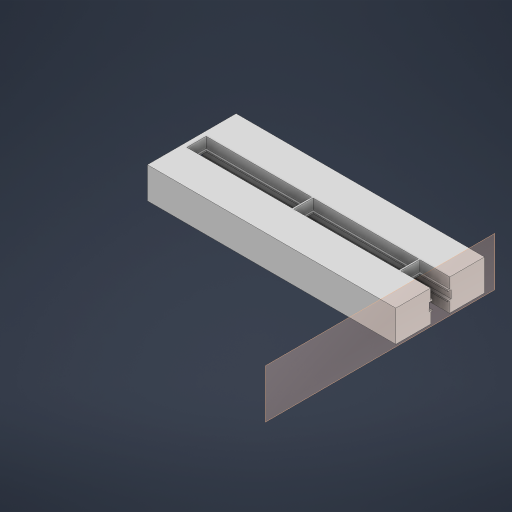
# Autodesk Inventor part: magnets nest half
Saved by Autodesk Inventor 2023 (Build 270158000, 158)
## iProperties
Created: 2023-08-23
Part Number: magnets nest half
Material: Generic
Document SubType Name: Modeling
Designer: f1a51
Density: 1 g/cm^3
Appearance: Default
Author: f1a51
Autodesk Inventor part; units mm, degrees
ref_plane "XZ Plane" through (0, 0, 0) normal (0, 1, 0) x (-1, 0, 0)
ref_plane "XY Plane" through (0, 0, 0) normal (0, 0, 1) x (1, 0, 0)
sketch "Sketch1" plane through (0, 0, 0) normal (1, 0, 0) x (0, 1, 0)
  line L0 (-6, -6) -> (6, -6)
  line L1 (6, -6) -> (6, 6)
  line L2 (6, 6) -> (-6, 6)
  line L3 (-6, 6) -> (-6, -6)
  line L4 (-6, -6) -> (6, 6) construction
  line L5 (6, -6) -> (-6, 6) construction
  line L6 (11, -40) -> (6, -40)
  line L7 (6, -40) -> (6, 40)
  line L8 (6, 40) -> (11, 40)
  line L9 (11, 40) -> (11, -40)
  line L10 (11, -40) -> (6, 40) construction
  line L11 (6, -40) -> (11, 40) construction
  line L12 (0, 24.7928) -> (0, 31.3359)
  line L13 (-11, -40) -> (-6, -40)
  line L14 (-6, -40) -> (-6, 40)
  line L15 (-6, 40) -> (-11, 40)
  line L16 (-11, 40) -> (-11, -40)
  line L17 (-11, -40) -> (-6, 40) construction
  line L18 (-6, -40) -> (-11, 40) construction
  line L19 (6, -21.3242) -> (2, -21.3242)
  line L20 (2, -21.3242) -> (2, -28.3242)
  line L21 (2, -28.3242) -> (6, -28.3242)
  line L22 (6, -28.3242) -> (6, -21.3242)
  line L23 (-6, -21.3242) -> (-2, -21.3242)
  line L24 (-2, -21.3242) -> (-2, -28.3242)
  line L25 (-2, -28.3242) -> (-6, -28.3242)
  line L26 (0, 0) -> (26.7242, 0)
  line L27 (6, 21.3242) -> (2, 21.3242)
  line L28 (2, 21.3242) -> (2, 28.3242)
  line L29 (2, 28.3242) -> (6, 28.3242)
  line L30 (-6, 21.3242) -> (-2, 21.3242)
  line L31 (-2, 21.3242) -> (-2, 28.3242)
  line L32 (-2, 28.3242) -> (-6, 28.3242)
  point P0 (8.5, 0)
  dimension "d0" = 12
  dimension "d1" = 12
  dimension "d2" = 80
  dimension "d3" = 5
  dimension "d4" = 0
  dimension "d5" = 0
  dimension "d6" = 4
  dimension "d7" = 7
  constraints: 66 end point, 16 symmetric about line, 6 parallel, 4 horizontal, 4 midpoint, 3 perpendicular, 1 point on line, 1 vertical
  measures "d0" distance of L1.end L2.end
  measures "d1" distance of L0.end L1.end
  measures "d2" distance of L8.end L6.start
  measures "d3" distance of L7.end L8.end
  measures "d4" vertical distance of L26.start point (8.5, 0)
  measures "d5" distance between parallel lines of L1 L7
  measures "d6" distance of L21.end L20.end
  measures "d7" distance of L20.end L19.end
extrude "Extrusion1" add sketch "Sketch1" along normal blind 290 contours L3 L2 L1 L0 | L1 L26 L9 L6 L7 | L1 L7 L8 L9 L26
sketch "Sketch3" plane through (0, 6, -40) normal (0, -1, 0) x (1, 0, 0)
  line L0 (290, 34) -> (290, 0) projected
  line L1 (290, 0) -> (290, 13.5)
  line L2 (290, 13.5) -> (288, 13.5)
  line L3 (288, 13.5) -> (288, 20.5)
  line L4 (288, 20.5) -> (248, 20.5)
  line L5 (248, 20.5) -> (248, 13.5)
  line L6 (248, 13.5) -> (288, 13.5)
  line L7 (248, 20.5) -> (247, 20.5)
  line L8 (247, 13.5) -> (247, 20.5)
  line L9 (247, 20.5) -> (207, 20.5)
  line L10 (207, 20.5) -> (207, 13.5)
  line L11 (207, 13.5) -> (247, 13.5)
  line L12 (207, 20.5) -> (206, 20.5)
  line L13 (206, 13.5) -> (206, 20.5)
  line L14 (206, 20.5) -> (166, 20.5)
  line L15 (166, 20.5) -> (166, 13.5)
  line L16 (166, 13.5) -> (206, 13.5)
  line L17 (166, 20.5) -> (165, 20.5)
  line L18 (165, 13.5) -> (165, 20.5)
  line L19 (165, 20.5) -> (125, 20.5)
  line L20 (125, 20.5) -> (125, 13.5)
  line L21 (125, 13.5) -> (165, 13.5)
  line L22 (125, 20.5) -> (124, 20.5)
  line L23 (124, 13.5) -> (124, 20.5)
  line L24 (124, 20.5) -> (84, 20.5)
  line L25 (84, 20.5) -> (84, 13.5)
  line L26 (84, 13.5) -> (124, 13.5)
  line L27 (84, 20.5) -> (83, 20.5)
  line L28 (83, 13.5) -> (83, 20.5)
  line L29 (83, 20.5) -> (43, 20.5)
  line L30 (43, 20.5) -> (43, 13.5)
  line L31 (43, 13.5) -> (83, 13.5)
  line L32 (43, 20.5) -> (42, 20.5)
  line L33 (42, 13.5) -> (42, 20.5)
  line L34 (42, 20.5) -> (2, 20.5)
  line L35 (2, 20.5) -> (2, 13.5)
  line L36 (2, 13.5) -> (42, 13.5)
  line L37 (0, 0) -> (290, 0) projected
  line L38 (0, 34) -> (290, 34) projected
  line L39 (0, 34) -> (0, 0) projected
  point P0 (0, 40)
  dimension "d15" = 13.5
  constraints: 72 end point, 15 perpendicular, 7 horizontal, 2 point on line
  measures "d15" distance of L0.end L1.end
extrude "Extrusion2" add sketch "Sketch3" along normal blind 12 separate body
sketch "Sketch4" plane through (0, 6, -40) normal (-1, 0, 0) x (0, 0, 1)
  line L0 (13.5, 0) -> (13.5, -12) projected
  line L1 (13.5, -12) -> (13.5, -8)
  line L2 (13.5, -8) -> (20.5, -8)
  line L3 (20.5, 0) -> (20.5, -12) projected
  line L4 (20.5, -8) -> (20.5, -4)
  line L5 (20.5, -4) -> (13.5, -4)
  line L6 (13.5, -8) -> (13.5, -4)
  point P0 (40, -6)
  dimension "d23" = 4
  dimension "d24" = 4
  constraints: 10 end point, 4 point on line, 3 perpendicular
  measures "d23" distance of L0.end L1.end
  measures "d24" distance of L2.end L4.end
extrude "Extrusion3" cut sketch "Sketch4" against normal blind 290 bodies 2
sketch "Sketch5" plane through (0, 6, -40) normal (-1, 0, 0) x (0, 0, 1)
  line L0 (20.5, -8) -> (13.5, -8) projected
  line L1 (13.5, -8) -> (13.5, -7.5)
  line L2 (13.5, -8) -> (13.5, -4) projected
  line L3 (13.5, -7.5) -> (20.5, -7.5)
  line L4 (20.5, -4) -> (20.5, -8) projected
  line L5 (20.5, -7.5) -> (20.5, -8)
  line L6 (13.5, -8) -> (13.5, -12) projected
  line L7 (20.5, -8) -> (13.5, -8)
  line L8 (13.5, -4) -> (20.5, -4) projected
  line L9 (13.5, -4) -> (13.5, -4.5)
  line L10 (13.5, -4.5) -> (20.5, -4.5)
  line L11 (20.5, 0) -> (20.5, -4) projected
  line L12 (20.5, -4.5) -> (20.5, -4)
  line L13 (13.5, 0) -> (13.5, -4) projected
  line L14 (20.5, -4) -> (13.5, -4)
  point P0 (40, -6)
  dimension "d27" = 0.5
  dimension "d28" = 0.5
  constraints: 16 end point, 4 point on line, 3 perpendicular, 1 collinear, 1 horizontal, 1 vertical
  measures "d27" distance of L0.end L1.end
  measures "d28" distance of L2.end L9.end
extrude "Extrusion4" add sketch "Sketch5" against normal blind 290 contours L0 L1 L3 L4 | L10 L2 L8 L4 bodies 2
sketch "Sketch6" plane through (248, -2, -26.5) normal (0, -1, 0) x (1, 0, 0)
  line L0 (-206, 7) -> (-206, 0)
  line L1 (-246, 7) -> (-206, 7)
  line L2 (-246, 0) -> (-246, 7)
  line L3 (-206, 0) -> (-246, 0)
  line L4 (-245.5, 0.5) -> (-245.5, 6.5)
  line L5 (-245.5, 6.5) -> (-206.5, 6.5)
  line L6 (-206.5, 6.5) -> (-206.5, 0.5)
  line L7 (-206.5, 0.5) -> (-245.5, 0.5)
  line L8 (-165, 7) -> (-165, 0)
  line L9 (-205, 7) -> (-165, 7)
  line L10 (-205, 0) -> (-205, 7)
  line L11 (-165, 0) -> (-205, 0)
  line L12 (-204.5, 0.5) -> (-204.5, 6.5)
  line L13 (-204.5, 6.5) -> (-165.5, 6.5)
  line L14 (-165.5, 6.5) -> (-165.5, 0.5)
  line L15 (-165.5, 0.5) -> (-204.5, 0.5)
  line L16 (-42, 7) -> (-42, 0)
  line L17 (-82, 7) -> (-42, 7)
  line L18 (-82, 0) -> (-82, 7)
  line L19 (-42, 0) -> (-82, 0)
  line L20 (-83, 7) -> (-83, 0)
  line L21 (-123, 7) -> (-83, 7)
  line L22 (-123, 0) -> (-123, 7)
  line L23 (-83, 0) -> (-123, 0)
  line L24 (-124, 7) -> (-124, 0)
  line L25 (-164, 7) -> (-124, 7)
  line L26 (-164, 0) -> (-164, 7)
  line L27 (-124, 0) -> (-164, 0)
  line L28 (-163.5, 0.5) -> (-163.5, 6.5)
  line L29 (-163.5, 6.5) -> (-124.5, 6.5)
  line L30 (-124.5, 6.5) -> (-124.5, 0.5)
  line L31 (-124.5, 0.5) -> (-163.5, 0.5)
  line L32 (-122.5, 0.5) -> (-122.5, 6.5)
  line L33 (-122.5, 6.5) -> (-83.5, 6.5)
  line L34 (-83.5, 6.5) -> (-83.5, 0.5)
  line L35 (-83.5, 0.5) -> (-122.5, 0.5)
  line L36 (-81.5, 0.5) -> (-81.5, 6.5)
  line L37 (-81.5, 6.5) -> (-42.5, 6.5)
  line L38 (-42.5, 6.5) -> (-42.5, 0.5)
  line L39 (-42.5, 0.5) -> (-81.5, 0.5)
  line L40 (0, 0) -> (0, 7)
  line L41 (40, 0) -> (0, 0)
  line L42 (40, 7) -> (40, 0)
  line L43 (0, 7) -> (40, 7)
  line L44 (-41, 0) -> (-41, 7)
  line L45 (-1, 0) -> (-41, 0)
  line L46 (-1, 7) -> (-1, 0)
  line L47 (-41, 7) -> (-1, 7)
  line L48 (-40.5, 0.5) -> (-40.5, 6.5)
  line L49 (-40.5, 6.5) -> (-1.5, 6.5)
  line L50 (-1.5, 6.5) -> (-1.5, 0.5)
  line L51 (-1.5, 0.5) -> (-40.5, 0.5)
  line L52 (0.5, 0.5) -> (0.5, 6.5)
  line L53 (0.5, 6.5) -> (39.5, 6.5)
  line L54 (39.5, 6.5) -> (39.5, 0.5)
  line L55 (39.5, 0.5) -> (0.5, 0.5)
  point P0 (-248, 26.5)
extrude "Extrusion5" cut sketch "Sketch6" against normal blind 6 contours L4 L5 L6 L7 | L12 L13 L14 L15 | L28 L29 L30 L31 | L32 L33 L34 L35 | L36 L37 L38 L39 | L48 L49 L50 L51 | L52 L53 L54 L55 bodies 2
sketch "Sketch7" plane through (290, 6, -6) normal (1, 0, 0) x (0, 0, -1)
  line L0 (20.5, -4.5) -> (21.2, -4.5)
  line L1 (21.2, -4.5) -> (21.2, -7.5)
  line L2 (21.2, -7.5) -> (20.5, -7.5)
  line L3 (20.5, -4.5) -> (13.5, -4.5) projected
  line L4 (20.5, -7.5) -> (20.5, -4.5)
  line L5 (13.5, -4.5) -> (12.8, -4.5)
  line L6 (12.8, -4.5) -> (12.8, -7.5)
  line L7 (12.8, -7.5) -> (13.5, -7.5)
  line L8 (13.5, -7.5) -> (13.5, -4.5)
  point P0 (-6, -6)
  dimension "d40" = 0.7
  dimension "d42" = 3
  dimension "d43" = 0.7
  dimension "d44" = 3
  constraints: 16 end point, 3 perpendicular, 2 horizontal, 1 vertical
  measures "d40" distance of L0.start L0.end
  measures "d42" distance of L0.end L1.end
  measures "d43" distance of L3.end L5.end
  measures "d44" distance of L5.end L6.end
extrude "Extrusion6" cut sketch "Sketch7" against normal blind 290 bodies 2
sketch "Sketch8" plane through (0, 6, -40) normal (0, 1, 0) x (1, 0, 0)
  line L0 (290, -34) -> (0, -34) projected
  line L1 (290, 0) -> (290, -34) projected
  line L2 (0, 0) -> (290, 0) projected
  line L3 (0, -34) -> (0, 0) projected
  line L4 (42, -20.5) -> (42, -13.5) projected
  line L5 (2, -20.5) -> (42, -20.5) projected
  line L6 (2, -13.5) -> (2, -20.5) projected
  line L7 (42, -13.5) -> (2, -13.5) projected
  line L8 (43, -20.5) -> (83, -20.5) projected
  line L9 (43, -13.5) -> (43, -20.5) projected
  line L10 (83, -13.5) -> (43, -13.5) projected
  line L11 (83, -20.5) -> (83, -13.5) projected
  line L12 (84, -20.5) -> (124, -20.5) projected
  line L13 (84, -13.5) -> (84, -20.5) projected
  line L14 (124, -13.5) -> (84, -13.5) projected
  line L15 (124, -20.5) -> (124, -13.5) projected
  line L16 (125, -20.5) -> (165, -20.5) projected
  line L17 (125, -13.5) -> (125, -20.5) projected
  line L18 (165, -13.5) -> (125, -13.5) projected
  line L19 (165, -20.5) -> (165, -13.5) projected
  line L20 (166, -20.5) -> (206, -20.5) projected
  line L21 (166, -13.5) -> (166, -20.5) projected
  line L22 (206, -13.5) -> (166, -13.5) projected
  line L23 (206, -20.5) -> (206, -13.5) projected
  line L24 (207, -20.5) -> (247, -20.5) projected
  line L25 (207, -13.5) -> (207, -20.5) projected
  line L26 (247, -13.5) -> (207, -13.5) projected
  line L27 (247, -20.5) -> (247, -13.5) projected
  line L28 (248, -20.5) -> (288, -20.5) projected
  line L29 (248, -13.5) -> (248, -20.5) projected
  line L30 (288, -13.5) -> (248, -13.5) projected
  line L31 (288, -20.5) -> (288, -13.5) projected
  line L32 (1.8, -13.3) -> (1.8, -20.7)
  line L33 (1.8, -20.7) -> (42.2, -20.7)
  line L34 (42.2, -20.7) -> (42.2, -13.3)
  line L35 (42.2, -13.3) -> (1.8, -13.3)
  line L36 (42.8, -13.3) -> (42.8, -20.7)
  line L37 (42.8, -20.7) -> (83.2, -20.7)
  line L38 (83.2, -20.7) -> (83.2, -13.3)
  line L39 (83.2, -13.3) -> (42.8, -13.3)
  line L40 (83.8, -13.3) -> (83.8, -20.7)
  line L41 (83.8, -20.7) -> (124.2, -20.7)
  line L42 (124.2, -20.7) -> (124.2, -13.3)
  line L43 (124.2, -13.3) -> (83.8, -13.3)
  line L44 (124.8, -13.3) -> (124.8, -20.7)
  line L45 (124.8, -20.7) -> (165.2, -20.7)
  line L46 (165.2, -20.7) -> (165.2, -13.3)
  line L47 (165.2, -13.3) -> (124.8, -13.3)
  line L48 (165.8, -13.3) -> (165.8, -20.7)
  line L49 (165.8, -20.7) -> (206.2, -20.7)
  line L50 (206.2, -20.7) -> (206.2, -13.3)
  line L51 (206.2, -13.3) -> (165.8, -13.3)
  line L52 (206.8, -13.3) -> (206.8, -20.7)
  line L53 (206.8, -20.7) -> (247.2, -20.7)
  line L54 (247.2, -20.7) -> (247.2, -13.3)
  line L55 (247.2, -13.3) -> (206.8, -13.3)
  line L56 (247.8, -13.3) -> (247.8, -20.7)
  line L57 (247.8, -20.7) -> (288.2, -20.7)
  line L58 (288.2, -20.7) -> (288.2, -13.3)
  line L59 (288.2, -13.3) -> (247.8, -13.3)
  point P0 (0, -40)
  dimension "d47" = 0.2
  dimension "d48" = 0.2
  dimension "d49" = 0.2
  dimension "d50" = 0.2
  dimension "d51" = 0.2
  dimension "d52" = 0.2
  dimension "d53" = 0.2
  constraints: 56 end point, 21 other
  measures "d47" distance between parallel lines of L7 L35
  measures "d48" distance between parallel lines of L10 L39
  measures "d49" distance between parallel lines of L14 L43
  measures "d50" distance between parallel lines of L18 L47
  measures "d51" distance between parallel lines of L22 L51
  measures "d52" distance between parallel lines of L26 L55
  measures "d53" distance between parallel lines of L30 L59
extrude "Extrusion7" cut sketch "Sketch8" against normal blind 4 contours L5 L6 L7 L4 | L35 L34 L33 L32 bodies 2
extrude "Extrusion8" cut sketch "Sketch8" against normal blind 4 contours L39 L38 L37 L36 | L43 L42 L41 L40 bodies 2
extrude "Extrusion9" cut sketch "Sketch8" against normal blind 4 contours L47 L46 L45 L44 | L51 L50 L49 L48 bodies 2
extrude "Extrusion10" cut sketch "Sketch8" against normal blind 4 contours L55 L54 L53 L52 | L59 L58 L57 L56 bodies 2
sketch "Sketch9" plane through (0, -6, -40) normal (0, -1, 0) x (1, 0, 0)
  line L0 (290, 34) -> (0, 34) projected
  line L1 (0, 34) -> (0, 0) projected
  line L2 (0, 0) -> (290, 0) projected
  line L3 (290, 0) -> (290, 34) projected
  line L4 (42, 20.5) -> (42, 13.5) projected
  line L5 (42, 13.5) -> (2, 13.5) projected
  line L6 (2, 13.5) -> (2, 20.5) projected
  line L7 (2, 20.5) -> (42, 20.5) projected
  line L8 (43, 20.5) -> (83, 20.5) projected
  line L9 (83, 20.5) -> (83, 13.5) projected
  line L10 (83, 13.5) -> (43, 13.5) projected
  line L11 (43, 13.5) -> (43, 20.5) projected
  line L12 (84, 20.5) -> (124, 20.5) projected
  line L13 (124, 20.5) -> (124, 13.5) projected
  line L14 (124, 13.5) -> (84, 13.5) projected
  line L15 (84, 13.5) -> (84, 20.5) projected
  line L16 (125, 20.5) -> (165, 20.5) projected
  line L17 (165, 20.5) -> (165, 13.5) projected
  line L18 (165, 13.5) -> (125, 13.5) projected
  line L19 (125, 13.5) -> (125, 20.5) projected
  line L20 (166, 20.5) -> (206, 20.5) projected
  line L21 (206, 20.5) -> (206, 13.5) projected
  line L22 (206, 13.5) -> (166, 13.5) projected
  line L23 (166, 13.5) -> (166, 20.5) projected
  line L24 (207, 20.5) -> (247, 20.5) projected
  line L25 (247, 20.5) -> (247, 13.5) projected
  line L26 (247, 13.5) -> (207, 13.5) projected
  line L27 (207, 13.5) -> (207, 20.5) projected
  line L28 (248, 20.5) -> (288, 20.5) projected
  line L29 (288, 20.5) -> (288, 13.5) projected
  line L30 (288, 13.5) -> (248, 13.5) projected
  line L31 (248, 13.5) -> (248, 20.5) projected
  line L32 (1.9, 13.4) -> (42.1, 13.4)
  line L33 (42.1, 13.4) -> (42.1, 20.6)
  line L34 (42.1, 20.6) -> (1.9, 20.6)
  line L35 (1.9, 20.6) -> (1.9, 13.4)
  line L36 (42.9, 13.4) -> (83.1, 13.4)
  line L37 (83.1, 13.4) -> (83.1, 20.6)
  line L38 (83.1, 20.6) -> (42.9, 20.6)
  line L39 (42.9, 20.6) -> (42.9, 13.4)
  line L40 (83.9, 13.4) -> (124.1, 13.4)
  line L41 (124.1, 13.4) -> (124.1, 20.6)
  line L42 (124.1, 20.6) -> (83.9, 20.6)
  line L43 (83.9, 20.6) -> (83.9, 13.4)
  line L44 (124.9, 13.4) -> (165.1, 13.4)
  line L45 (165.1, 13.4) -> (165.1, 20.6)
  line L46 (165.1, 20.6) -> (124.9, 20.6)
  line L47 (124.9, 20.6) -> (124.9, 13.4)
  line L48 (165.9, 13.4) -> (206.1, 13.4)
  line L49 (206.1, 13.4) -> (206.1, 20.6)
  line L50 (206.1, 20.6) -> (165.9, 20.6)
  line L51 (165.9, 20.6) -> (165.9, 13.4)
  line L52 (206.9, 13.4) -> (247.1, 13.4)
  line L53 (247.1, 13.4) -> (247.1, 20.6)
  line L54 (247.1, 20.6) -> (206.9, 20.6)
  line L55 (206.9, 20.6) -> (206.9, 13.4)
  line L56 (247.9, 13.4) -> (288.1, 13.4)
  line L57 (288.1, 13.4) -> (288.1, 20.6)
  line L58 (288.1, 20.6) -> (247.9, 20.6)
  line L59 (247.9, 20.6) -> (247.9, 13.4)
  point P0 (0, 40)
  dimension "d62" = 0.1
  dimension "d63" = 0.1
  dimension "d64" = 0.1
  dimension "d65" = 0.1
  dimension "d66" = 0.1
  dimension "d67" = 0.1
  dimension "d68" = 0.1
  constraints: 56 end point, 21 other
  measures "d62" distance between parallel lines of L5 L32
  measures "d63" distance between parallel lines of L10 L36
  measures "d64" distance between parallel lines of L14 L40
  measures "d65" distance between parallel lines of L18 L44
  measures "d66" distance between parallel lines of L22 L48
  measures "d67" distance between parallel lines of L26 L52
  measures "d68" distance between parallel lines of L30 L56
extrude "Extrusion11" cut sketch "Sketch9" against normal blind 4 contours L55 L54 L53 L52 | L59 L58 L57 L56 bodies 2
extrude "Extrusion12" cut sketch "Sketch9" against normal blind 4 contours L47 L46 L45 L44 | L51 L50 L49 L48 bodies 2
extrude "Extrusion13" cut sketch "Sketch9" against normal blind 4 contours L39 L38 L37 L36 | L43 L42 L41 L40 bodies 2
extrude "Extrusion14" cut sketch "Sketch9" against normal blind 4 contours L35 L34 L33 L32 bodies 2
ref_plane "Work Plane1" through (95.25, 0, 0) normal (1, 0, 0) x (0, 1, 0)
split "Split1" plane through (95.25, 0, 0) removes the side toward (1, 0, 0) bodies 2
body "Solid1"
body "Solid2"
